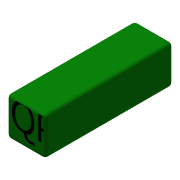
# Autodesk Inventor part: Container 2 2 5 colored color 2
Saved by Autodesk Inventor 2015 (Build 190159000, 159)
## iProperties
Created: 2015-03-07
Part Number: Container 2 2 5 colored color 2
Material: Generic
Document SubType Name: Modeling
Designer: Vukica
Density: 1 g/cm^3
Appearance: Dark Green
Author: Vukica
Autodesk Inventor part; units mm, degrees
ref_plane "YZ Plane" through (0, 0, 0) normal (1, 0, 0) x (0, 1, 0)
ref_plane "XZ Plane" through (0, 0, 0) normal (0, 1, 0) x (-1, 0, 0)
ref_plane "XY Plane" through (0, 0, 0) normal (0, 0, 1) x (1, 0, 0)
sketch "Sketch1" plane through (0, 0, 0) normal (0, 0, 1) x (1, 0, 0)
  line L0 (0, 0) -> (38.1, 0)
  line L1 (38.1, 0) -> (38.1, 38.1)
  line L2 (38.1, 38.1) -> (0, 38.1)
  line L3 (0, 38.1) -> (0, 0)
  dimension "d0" = 38.1
  dimension "d1" = 38.1
  constraints: 8 end point, 2 parallel, 1 horizontal, 1 perpendicular
  measures "d0" distance of L1.end L2.end
  measures "d1" distance of L2.end L0.start
extrude "Extrusion1" add sketch "Sketch1" along normal blind 127
sketch "Sketch2" plane through (0, 0, 127) normal (0, 0, 1) x (1, 0, 0)
  line L0 (0.6032, 32.2606) -> (46.9983, 32.2606) construction
  line L1 (46.9983, 32.2606) -> (46.9983, -9.6319) construction
  line L2 (46.9983, -9.6319) -> (0.6032, -9.6319) construction
  line L3 (0.6032, -9.6319) -> (0.6032, 32.2606) construction
  spline S0 degree 2 poles (19.54, 6.5395) (18.799, 6.3584) (17.1852, 6.1608) (16.3784, 6.1608) knots 0 0 0 1 2 2 2
  spline S1 degree 2 poles (16.3784, 6.1608) (14.0895, 6.1608) (11.2407, 8.7131) (11.109, 11.0843) knots 0 0 0 1 2 2 2
  spline S2 degree 2 poles (11.109, 11.0843) (10.9279, 11.0843) (10.615, 11.0843) (10.4833, 11.0843) knots 0 0 0 1 2 2 2
  spline S3 degree 2 poles (10.4833, 11.0843) (8.4249, 11.0843) (5.1151, 12.484) (3.9295, 13.8508) knots 0 0 0 1 2 2 2
  spline S4 degree 2 poles (3.9295, 13.8508) (2.7604, 15.201) (1.5089, 19.1531) (1.5089, 21.656) knots 0 0 0 1 2 2 2
  spline S5 degree 2 poles (1.5089, 21.656) (1.5089, 24.2248) (2.7768, 28.111) (3.946, 29.4942) knots 0 0 0 1 2 2 2
  spline S6 degree 2 poles (3.946, 29.4942) (5.1316, 30.8609) (8.4414, 32.2606) (10.4833, 32.2606) knots 0 0 0 1 2 2 2
  spline S7 degree 2 poles (10.4833, 32.2606) (12.5581, 32.2606) (15.8844, 30.8115) (17.037, 29.4942) knots 0 0 0 1 2 2 2
  spline S8 degree 2 poles (17.037, 29.4942) (18.1897, 28.1604) (19.4741, 24.1919) (19.4741, 21.656) knots 0 0 0 1 2 2 2
  spline S9 degree 2 poles (19.4741, 21.656) (19.4741, 17.704) (16.3948, 12.5664) (13.7108, 11.6607) knots 0 0 0 1 2 2 2
  spline S10 degree 2 poles (13.7108, 11.6607) (13.7766, 10.9032) (14.1718, 9.6847) (14.4847, 9.3389) knots 0 0 0 1 2 2 2
  spline S11 degree 2 poles (14.4847, 9.3389) (14.8634, 8.9107) (15.9008, 8.5155) (16.823, 8.5155) knots 0 0 0 1 2 2 2
  spline S12 degree 2 poles (16.823, 8.5155) (17.3664, 8.5155) (18.8484, 8.8613) (19.1777, 8.9931) knots 0 0 0 1 2 2 2
  line L4 (19.1777, 8.9931) -> (19.54, 8.9931)
  line L5 (19.54, 8.9931) -> (19.54, 6.5395)
  spline S13 degree 2 poles (16.6583, 21.656) (16.6583, 23.6814) (15.7856, 26.7936) (14.9952, 27.8146) knots 0 0 0 1 2 2 2
  spline S14 degree 2 poles (14.9952, 27.8146) (14.1883, 28.8685) (11.9159, 29.9223) (10.4997, 29.9223) knots 0 0 0 1 2 2 2
  spline S15 degree 2 poles (10.4997, 29.9223) (9.0342, 29.9223) (6.8276, 28.9014) (5.9878, 27.8146) knots 0 0 0 1 2 2 2
  spline S16 degree 2 poles (5.9878, 27.8146) (5.181, 26.7772) (4.3247, 23.632) (4.3247, 21.656) knots 0 0 0 1 2 2 2
  spline S17 degree 2 poles (4.3247, 21.656) (4.3247, 17.6546) (7.6839, 13.3897) (10.4997, 13.3897) knots 0 0 0 1 2 2 2
  spline S18 degree 2 poles (10.4997, 13.3897) (13.3156, 13.3897) (16.6583, 17.6546) (16.6583, 21.656) knots 0 0 0 1 2 2 2
  line L6 (38.1639, 11.5125) -> (34.6565, 11.5125)
  line L7 (34.6565, 11.5125) -> (28.2345, 19.5977)
  line L8 (28.2345, 19.5977) -> (25.1387, 19.5977)
  line L9 (25.1387, 19.5977) -> (25.1387, 11.5125)
  line L10 (25.1387, 11.5125) -> (22.4381, 11.5125)
  line L11 (22.4381, 11.5125) -> (22.4381, 31.8325)
  line L12 (22.4381, 31.8325) -> (27.6746, 31.8325)
  spline S19 degree 2 poles (27.6746, 31.8325) (29.4201, 31.8325) (31.7748, 31.4537) (32.8452, 30.7621) knots 0 0 0 1 2 2 2
  spline S20 degree 2 poles (32.8452, 30.7621) (33.9155, 30.0705) (35.1505, 27.9134) (35.1505, 26.3161) knots 0 0 0 1 2 2 2
  spline S21 degree 2 poles (35.1505, 26.3161) (35.1505, 24.0931) (32.8781, 21.0797) (30.935, 20.3551) knots 0 0 0 1 2 2 2
  line L13 (30.935, 20.3551) -> (38.1639, 11.5125)
  spline S22 degree 2 poles (32.3347, 26.102) (32.3347, 26.9913) (31.7089, 28.358) (31.0503, 28.8026) knots 0 0 0 1 2 2 2
  spline S23 degree 2 poles (31.0503, 28.8026) (30.4739, 29.1813) (28.9425, 29.4942) (27.8228, 29.4942) knots 0 0 0 1 2 2 2
  line L14 (27.8228, 29.4942) -> (25.1387, 29.4942)
  line L15 (25.1387, 29.4942) -> (25.1387, 21.8536)
  line L16 (25.1387, 21.8536) -> (27.5099, 21.8536)
  spline S24 degree 2 poles (27.5099, 21.8536) (28.6791, 21.8536) (30.5398, 22.2653) (31.182, 22.9075) knots 0 0 0 1 2 2 2
  spline S25 degree 2 poles (31.182, 22.9075) (31.7748, 23.4674) (32.3347, 25.0482) (32.3347, 26.102) knots 0 0 0 1 2 2 2
  point P0 (0, 0)
  constraints: 2 other
fillet "Fillet1" radius 3.175 4 edges at (38.1, 38.1, 63.5) (0, 38.1, 63.5) (0, 0, 63.5) (38.1, 0, 63.5)
fillet "Fillet2" radius 3.175 16 edges at (37.1701, 0.9299, 127) (38.1, 19.05, 127) (37.1701, 37.1701, 127) (19.05, 38.1, 127) (0.9299, 37.1701, 127) (0, 19.05, 127) (0.9299, 0.9299, 127) (19.05, 0, 127) (37.1701, 0.9299, 0) (38.1, 19.05, 0) (37.1701, 37.1701, 0) (19.05, 38.1, 0) (0.9299, 37.1701, 0) (0, 19.05, 0) (0.9299, 0.9299, 0) (19.05, 0, 0)
extrude "Extrusion3" cut sketch "Sketch2" against normal blind 0.254
body "Solid1"
